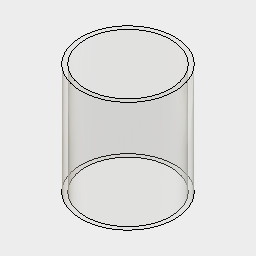
Acryllic Tube (Autodesk Fusion 360 design; units mm, degrees)
Autodesk Fusion 360 part; units mm, degrees
sketch "Sketch1" plane through (0, 0, 0) normal (0, 1, 0) x (1, 0, 0)
  circle A0 centre (0, 0) radius 27.5
  circle A1 centre (0, 0) radius 25
  dimension "d1" = 55
  measures "d1" diameter of A0
extrude "Extrude1" add sketch "Sketch1" along normal blind 65
